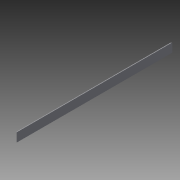
# Autodesk Inventor part: body_outer_L
Saved by Autodesk Inventor 2015 (Build 190159000, 159)
## iProperties
Created: 2017-09-26
Part Number: body_outer_L
Material: Generic
Document SubType Name: Modeling
Designer: Anshul
Density: 1 g/cm^3
Appearance: Default
Author: Anshul
Autodesk Inventor part; units mm, degrees
ref_plane "YZ Plane" through (0, 0, 0) normal (1, 0, 0) x (0, 1, 0)
ref_plane "XZ Plane" through (0, 0, 0) normal (0, 1, 0) x (-1, 0, 0)
ref_plane "XY Plane" through (0, 0, 0) normal (0, 0, 1) x (1, 0, 0)
sketch "Sketch1" plane through (0, 0, 0) normal (0, 1, 0) x (-1, 0, 0)
  line L0 (0, 0) -> (0, -650)
  line L1 (0, -650) -> (650, -650)
  line L2 (650, -650) -> (650, 0)
  line L3 (650, 0) -> (0, 0)
  line L4 (0, 0) -> (3, 0)
  line L5 (3, -3) -> (3, -647)
  line L6 (3, -650) -> (0, -650)
  line L7 (0, -650) -> (0, -647)
  line L8 (650, -647) -> (650, -650)
  line L9 (650, -650) -> (647, -650)
  line L10 (647, -650) -> (647, 0)
  line L11 (647, 0) -> (650, 0)
  line L12 (650, 0) -> (650, -3)
  line L13 (0, -3) -> (0, 0)
  line L14 (0, 0) -> (0, -37)
  line L15 (650, -37) -> (650, 0)
  line L16 (650, 0) -> (613, 0)
  line L17 (613, 0) -> (613, -650)
  line L18 (613, -650) -> (650, -650)
  line L19 (650, -650) -> (650, -613)
  line L20 (0, -613) -> (0, -650)
  line L21 (0, -650) -> (37, -650)
  line L22 (37, 0) -> (0, 0)
  line L23 (3, -147.3087) -> (3, -94.9828)
  line L24 (147.3087, -3) -> (94.9828, -3)
  circle A0 centre (16.1109, -108.0348) radius 3
  line L25 (0, -650) -> (3, -650)
  line L26 (0, -647) -> (0, -650)
  line L27 (0, -650) -> (0, -613)
  line L28 (37, -650) -> (0, -650)
  line L29 (3, -502.6913) -> (3, -555.0172)
  line L30 (147.3087, -647) -> (94.9828, -647)
  circle A1 centre (16.1109, -541.9652) radius 3
  line L31 (37, -650) -> (37, -37)
  line L32 (37, -3) -> (37, 0)
  line L33 (650, -3) -> (34.9546, -3)
  line L34 (34.9546, -647) -> (650, -647)
  line L35 (37, -37) -> (0, 0)
  line L36 (37, -613) -> (0, -650)
  line L37 (0, -650) -> (3, -647)
  line L38 (3, -647) -> (3, -3)
  line L39 (3, -3) -> (0, 0)
  line L40 (3, -325) -> (3, -458)
  line L41 (3, -458) -> (20, -458)
  line L42 (3, -325) -> (3, -192)
  line L43 (3, -192) -> (20, -192)
  circle A2 centre (20, -192) radius 3
  circle A3 centre (20, -458) radius 3
  line L44 (325, -650) -> (192, -650)
  line L45 (192, -650) -> (192, -630)
  circle A4 centre (192, -630) radius 3
  line L46 (3, -458) -> (3, -475)
  line L47 (3, -475) -> (647, -475)
  line L48 (3, -475) -> (3, -478)
  line L49 (3, -478) -> (647, -478)
  line L50 (192, -630) -> (175, -630)
  line L51 (192, -630) -> (209, -630)
  line L52 (209, -630) -> (209, -478)
  line L53 (175, -630) -> (175, -478)
  point P0 (37, -647)
  dimension "d0" = 650
  dimension "d1" = 650
  dimension "d2" = 650
  dimension "d3" = 3
  dimension "d4" = 650
  dimension "d5" = 3
  dimension "d6" = 3
  dimension "d7" = 650
  dimension "d8" = 3
  dimension "d9" = 650
  dimension "d10" = 37
  dimension "d12" = 37
  dimension "d13" = 650
  dimension "d14" = 37
  dimension "d15" = 650
  dimension "d16" = 37
  dimension "d28" = 6
  dimension "d33" = 133
  dimension "d34" = 17
  dimension "d35" = 133
  dimension "d36" = 17
  dimension "d37" = 6
  dimension "d38" = 6
  dimension "d41" = 133
  dimension "d42" = 20
  dimension "d43" = 6
  dimension "d44" = 17
  dimension "d45" = 3
  dimension "d46" = 17
  dimension "d47" = 17
  constraints: 108 end point, 32 point on line, 12 perpendicular, 7 collinear, 5 centre point, 3 coincident, 2 midpoint, 2 vertical, 1 parallel
  measures "d0" distance of L0.start L0.end
  measures "d1" distance of L0.end L1.end
  measures "d2" distance of L1.end L2.end
  measures "d3" distance of L0.start L4.end
  measures "d4" distance of L4.end L6.start
  measures "d5" distance of L0.end L7.end
  measures "d6" distance of L1.end L9.end
  measures "d7" distance of L9.end L10.end
  measures "d8" distance of L2.end L12.end
  measures "d9" distance of L12.end L13.start
  measures "d10" distance of L0.start L14.end
  measures "d12" distance of L2.end L16.end
  measures "d13" distance of L16.end L17.end
  measures "d14" distance of L1.end L19.end
  measures "d15" distance of L19.end L20.start
  measures "d16" distance of L0.end L21.end
  measures "d28" diameter of A0
  measures "d33" distance of L40.start L40.end
  measures "d34" distance of L40.end L41.end
  measures "d35" distance of L40.start L42.end
  measures "d36" distance of L42.end L43.end
  measures "d37" diameter of A2
  measures "d38" diameter of A3
  measures "d41" distance of L44.start L44.end
  measures "d42" distance of L44.end L45.end
  measures "d43" diameter of A4
  measures "d44" distance of L40.end L46.end
  measures "d45" distance of L46.end L48.end
  measures "d46" distance of L50.start L50.end
  measures "d47" distance of L50.start L51.end
extrude "Extrusion1" add sketch "Sketch1" along normal blind 3 contours L35 L5 L36 L0 | A2 | A3 | L35 L31 L47 L5 | L31 L49 L5 L47 | L31 L36 L5 L49
extrude "Extrusion2" add sketch "Sketch1" along normal blind 37 contours L35 L5 L36 L0
extrude "Extrusion3" cut sketch "Sketch1" along normal blind 3 contours A2 | A3
body "Solid1"
